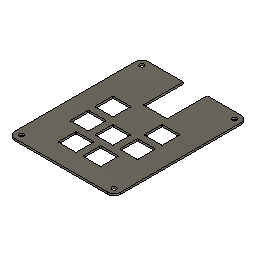
Macropad_Top_Cover (Autodesk Fusion 360 design; units mm, degrees)
Autodesk Fusion 360 part; units mm, degrees
sketch "plate-2025-12-07T05_26_02.564Z" plane through (0, 0, 0) normal (0, 0, 1) x (1, 0, 0)
  line L0 (3.025, -2.525) -> (16.025, -2.525)
  line L1 (3.025, -16.525) -> (16.025, -16.525)
  line L2 (2.525, -3.025) -> (2.525, -16.025)
  line L3 (16.525, -3.025) -> (16.525, -16.025)
  arc A0 (3.025, -2.525) -> (2.525, -3.025) centre (3.025, -3.025) ccw
  arc A1 (16.525, -3.025) -> (16.025, -2.525) centre (16.025, -3.025) ccw
  arc A2 (2.525, -16.025) -> (3.025, -16.525) centre (3.025, -16.025) ccw
  arc A3 (16.025, -16.525) -> (16.525, -16.025) centre (16.025, -16.025) ccw
  line L4 (41.125, -2.525) -> (54.125, -2.525)
  line L5 (41.125, -16.525) -> (54.125, -16.525)
  line L6 (40.625, -3.025) -> (40.625, -16.025)
  line L7 (54.625, -3.025) -> (54.625, -16.025)
  arc A4 (41.125, -2.525) -> (40.625, -3.025) centre (41.125, -3.025) ccw
  arc A5 (54.625, -3.025) -> (54.125, -2.525) centre (54.125, -3.025) ccw
  arc A6 (40.625, -16.025) -> (41.125, -16.525) centre (41.125, -16.025) ccw
  arc A7 (54.125, -16.525) -> (54.625, -16.025) centre (54.125, -16.025) ccw
  line L8 (3.025, -21.575) -> (16.025, -21.575)
  line L9 (3.025, -35.575) -> (16.025, -35.575)
  line L10 (2.525, -22.075) -> (2.525, -35.075)
  line L11 (16.525, -22.075) -> (16.525, -35.075)
  arc A8 (3.025, -21.575) -> (2.525, -22.075) centre (3.025, -22.075) ccw
  arc A9 (16.525, -22.075) -> (16.025, -21.575) centre (16.025, -22.075) ccw
  arc A10 (2.525, -35.075) -> (3.025, -35.575) centre (3.025, -35.075) ccw
  arc A11 (16.025, -35.575) -> (16.525, -35.075) centre (16.025, -35.075) ccw
  line L12 (22.075, -21.575) -> (35.075, -21.575)
  line L13 (22.075, -35.575) -> (35.075, -35.575)
  line L14 (21.575, -22.075) -> (21.575, -35.075)
  line L15 (35.575, -22.075) -> (35.575, -35.075)
  arc A12 (22.075, -21.575) -> (21.575, -22.075) centre (22.075, -22.075) ccw
  arc A13 (35.575, -22.075) -> (35.075, -21.575) centre (35.075, -22.075) ccw
  arc A14 (21.575, -35.075) -> (22.075, -35.575) centre (22.075, -35.075) ccw
  arc A15 (35.075, -35.575) -> (35.575, -35.075) centre (35.075, -35.075) ccw
  line L16 (41.125, -21.575) -> (54.125, -21.575)
  line L17 (41.125, -35.575) -> (54.125, -35.575)
  line L18 (40.625, -22.075) -> (40.625, -35.075)
  line L19 (54.625, -22.075) -> (54.625, -35.075)
  arc A16 (41.125, -21.575) -> (40.625, -22.075) centre (41.125, -22.075) ccw
  arc A17 (54.625, -22.075) -> (54.125, -21.575) centre (54.125, -22.075) ccw
  arc A18 (40.625, -35.075) -> (41.125, -35.575) centre (41.125, -35.075) ccw
  arc A19 (54.125, -35.575) -> (54.625, -35.075) centre (54.125, -35.075) ccw
  line L20 (12.55, -40.625) -> (25.55, -40.625)
  line L21 (12.55, -54.625) -> (25.55, -54.625)
  line L22 (12.05, -41.125) -> (12.05, -54.125)
  line L23 (26.05, -41.125) -> (26.05, -54.125)
  arc A20 (12.55, -40.625) -> (12.05, -41.125) centre (12.55, -41.125) ccw
  arc A21 (26.05, -41.125) -> (25.55, -40.625) centre (25.55, -41.125) ccw
  arc A22 (12.05, -54.125) -> (12.55, -54.625) centre (12.55, -54.125) ccw
  arc A23 (25.55, -54.625) -> (26.05, -54.125) centre (25.55, -54.125) ccw
  line L24 (31.6, -40.625) -> (44.6, -40.625)
  line L25 (31.6, -54.625) -> (44.6, -54.625)
  line L26 (31.1, -41.125) -> (31.1, -54.125)
  line L27 (45.1, -41.125) -> (45.1, -54.125)
  arc A24 (31.6, -40.625) -> (31.1, -41.125) centre (31.6, -41.125) ccw
  arc A25 (45.1, -41.125) -> (44.6, -40.625) centre (44.6, -41.125) ccw
  arc A26 (31.1, -54.125) -> (31.6, -54.625) centre (31.6, -54.125) ccw
  arc A27 (44.6, -54.625) -> (45.1, -54.125) centre (44.6, -54.125) ccw
  line L28 (-11.896, 34.298) -> (70.017, 34.298)
  line L29 (70.017, 34.298) -> (70.017, -69.046)
  line L30 (70.017, -69.046) -> (-11.896, -69.046)
  line L31 (-11.896, -69.046) -> (-11.896, 34.298)
  line L32 (20.315, 34.298) -> (38.815, 34.298)
  line L33 (38.815, 34.298) -> (38.815, 3.298)
  line L34 (38.815, 3.298) -> (20.315, 3.298)
  line L35 (20.315, 3.298) -> (20.315, 34.298)
  circle A28 centre (-6.896, 29.298) radius 1.7
  circle A29 centre (65.017, 29.298) radius 1.7
  circle A30 centre (-6.896, -64.046) radius 1.7
  circle A31 centre (65.017, -64.046) radius 1.7
  dimension "d1" = 81.913
  dimension "d2" = 103.344
  dimension "d3" = 23.946
  dimension "d4" = 14.421
  dimension "d5" = 18.5
  dimension "d6" = 31
  dimension "d7" = 32.211
  dimension "d8" = 3.4
  dimension "d9" = 3.4
  dimension "d10" = 3.4
  dimension "d11" = 3.4
  dimension "d12" = 5
  dimension "d13" = 5
  dimension "d14" = 5
  dimension "d15" = 5
  dimension "d16" = 5
  dimension "d17" = 5
  dimension "d18" = 5
  dimension "d19" = 5
  constraint horizontal L28
  constraint vertical L29
  constraint horizontal L30
  constraint vertical L31
  constraint horizontal L32
  constraint vertical L33
  constraint horizontal L34
  constraint vertical L35
  constraint coincident L28 L32.start
  measures "d1" distance of L28.start L28.end
  measures "d2" distance of L28.start L30.end
  measures "d3" distance of L22 L31
  measures "d4" distance of L21 L30
  measures "d5" distance of L32.start L32.end
  measures "d6" distance of L32.start L34.end
  measures "d7" distance of L31 L35
  measures "d8" diameter of A28
  measures "d9" diameter of A29
  measures "d10" diameter of A30
  measures "d11" diameter of A31
  measures "d12" distance of L31 A28.centre
  measures "d13" distance of L29 A29.centre
  measures "d14" distance of L30 A31.centre
  measures "d15" distance of L29 A31.centre
  measures "d16" distance of L28 A29.centre
  measures "d17" distance of L28 A28.centre
  measures "d18" distance of L30 A30.centre
  measures "d19" distance of L31 A30.centre
extrude "Extrude1" add sketch "plate-2025-12-07T05_26_02.564Z" along normal blind 1.5 contours L28 L29 L30 L31 L33 L34 L35
fillet "Fillet1" radius 5 4 edges at (-11.896, -69.046, 0.75) (70.017, -69.046, 0.75) (70.017, 34.298, 0.75) (-11.896, 34.298, 0.75)
